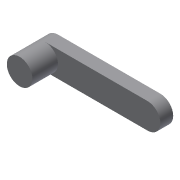
# Autodesk Inventor part: sliderarm
Saved by Autodesk Inventor 2022 (Build 260148000, 148)
## iProperties
Shininess: 64.0
Length Units: 11269
Angle Units: 11279
Time Units: 11290
Mass Units: 11283
Length Display Precision: 3
Angle Display Precision: 2
Created: 2001-12-31
Part Number: sliderarm
Document SubType Name: Modeling
Designer: Administrator
Density: 1 g/cm^3
Material: Generic
Appearance: Default
Density: 0.0
Volumn: 0.0
Area: 0.0
PropertySet Name: Model Information
Control State: 0
Master: False
Checked Out: False
Author: Administrator
Autodesk Inventor part; units mm, degrees
ref_plane "YZ Plane" through (0, 0, 0) normal (1, 0, 0) x (0, 1, 0)
ref_plane "XZ Plane" through (0, 0, 0) normal (0, 1, 0) x (-1, 0, 0)
ref_plane "XY Plane" through (0, 0, 0) normal (0, 0, 1) x (1, 0, 0)
sketch "Sketch1" plane through (0, 0, 0) normal (0, 0, 1) x (1, 0, 0)
  line L0 (-14.7447, 9.502) -> (36.0553, 9.502)
  line L1 (42.4053, 3.152) -> (42.4053, 3.152)
  line L2 (36.0553, -3.198) -> (-14.7447, -3.198)
  line L3 (-21.0947, 3.152) -> (-21.0947, 3.152)
  arc A0 (-14.7447, 9.502) -> (-21.0947, 3.152) centre (-14.7447, 3.152) ccw
  arc A1 (-21.0947, 3.152) -> (-14.7447, -3.198) centre (-14.7447, 3.152) ccw
  arc A2 (42.4053, 3.152) -> (36.0553, 9.502) centre (36.0553, 3.152) ccw
  arc A3 (36.0553, -3.198) -> (42.4053, 3.152) centre (36.0553, 3.152) ccw
  point P0 (-21.0947, 9.502)
  point P1 (-21.0947, -3.198)
  dimension "d0" = 12.7
  dimension "d1" = 6.35
  dimension "d2" = 50.8
  constraints: 8 end point, 8 point on circle, 8 tangent, 4 centre point, 4 point on line, 3 equal radius, 2 parallel, 1 horizontal, 1 perpendicular
  measures "d0" distance of point (-21.095, -3.198) point (-21.095, 9.502)
  measures "d1" radius of A0
  measures "d2" distance of L0.start L0.end
extrude "Extrusion1" add sketch "Sketch1" along normal blind 6.35
sketch "Sketch3" plane through (0, 0, 6.35) normal (0, 0, 1) x (1, 0, 0)
  arc A0 (-14.7447, 9.502) -> (-14.7447, -3.198) centre (-14.7447, 3.152) ccw projected
  circle A1 centre (-14.7447, 3.152) radius 6.35
  dimension "d12" = 12.7
  constraints: 1 centre point, 1 coincident
  measures "d12" diameter of A1
extrude "Extrusion2" add sketch "Sketch3" along normal blind 12.7
body "Solid1"
